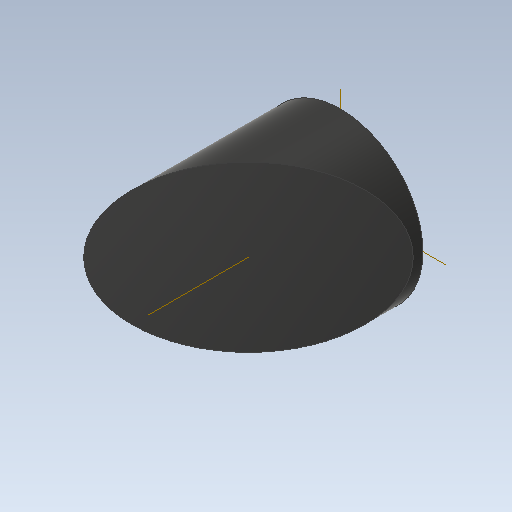
# Autodesk Inventor part: trzymadlo
Saved by Autodesk Inventor 2020 (Build 240168000, 168)
## iProperties
Created: 2019-05-25
Part Number: trzymadlo
Material: ABS Plastic
Document SubType Name: Modeling
Designer: Esterka
Density: 1.06 g/cm^3
Appearance: Smooth - White
Author: Esterka
Autodesk Inventor part; units mm, degrees
ref_plane "YZ Plane" through (0, 0, 0) normal (1, 0, 0) x (0, 1, 0)
ref_plane "XY Plane" through (0, 0, 0) normal (0, 0, 1) x (1, 0, 0)
sketch "Sketch1" plane through (0, 0, 0) normal (0, 0, 1) x (1, 0, 0)
  circle A0 centre (0, 0) radius 17
  dimension "d0" = 34
  constraints: 1 centre point, 1 coincident
  measures "d0" diameter of A0
extrude "Extrusion1" add sketch "Sketch1" along normal blind 36
sketch "Sketch2" plane through (0, 0, 0) normal (0, 1, 0) x (-1, 0, 0)
  line L0 (17, 36) -> (-17, 36) projected
  line L1 (17, 36) -> (-17.212, 1.788)
  point P0 (0, 0)
  dimension "d3" = 45
  constraints: 2 end point
  measures "d3" angle of L0 L1
ref_plane "Work Plane1" through (-17, 0, 36) normal (0.7071, 0, 0.7071) x (0.7071, 0, -0.7071)
split "Split2" plane through (-17, 0, 36) removes the side toward (0.7071, 0, 0.7071)
sketch "Sketch3" plane through (0, 0, 0) normal (0, 0, -1) x (-1, 0, 0)
  circle A0 centre (0, 0) radius 12
  circle A1 centre (6.0165, -10.3828) radius 2.5
  circle A2 centre (5.9835, 10.4018) radius 2.5
  circle A3 centre (-12, -0.0191) radius 2.5
  dimension "d5" = 24
  dimension "d6" = 5
  dimension "d9" = 360
  constraints: 3 centre point, 1 coincident, 10 other
  measures "d6" diameter of A1
extrude "Extrusion2" cut sketch "Sketch3" against normal blind 3 contours A2 A0 | A0 A2 | A1 A0 | A0 A1 | A3 A0 | A0 A3
sketch "Sketch4" plane through (0, 0, 0) normal (0, 0, -1) x (-1, 0, 0)
  point P0 (0, -12)
body "Solid1"
